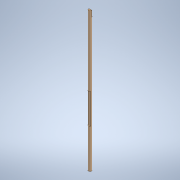
# Autodesk Inventor part: Wheel Shaft 125mm
Saved by Autodesk Inventor 2021.1 (Build 251245010, 245A)
## iProperties
Created: 2025-09-16
Material: Bronze, Soft Tin
Document SubType Name: Modeling
Designer: SD
Density: 8.874 g/cm^3
Appearance: Brindle
Mass: 8.09145 g
Surface Area: 13.019 cm^2
Volume: 0.911816 cm^3
Project: Automatic Tea Steeping mechanism
Part Number: Wheel Shaft 125mm
Length: 139.500 mm
BOM-Mass: 0.00809
BOM-Area: 0.001
Diameter: 3.000 mm
Author: SD
Title: Wheel Shaft 125mm
Autodesk Inventor part; units mm, degrees
ref_plane "YZ Plane" through (0, 0, 0) normal (1, 0, 0) x (0, 1, 0)
ref_plane "XZ Plane" through (0, 0, 0) normal (0, 1, 0) x (-1, 0, 0)
ref_plane "XY Plane" through (0, 0, 0) normal (0, 0, 1) x (1, 0, 0)
sketch "Sketch4" plane through (0, 0, 0) normal (0, 1, 0) x (-1, 0, 0)
  circle A0 centre (0, 0) radius 1.5
  constraints: 1 centre point, 1 coincident, 1 other
extrude "Extrusion2" add sketch "Sketch4" along normal mid plane 139.5
sketch "Sketch13" plane through (0, 0, 0) normal (1, 0, 0) x (0, 1, 0)
  line L0 (70.3754, -0.5) -> (63.75, -0.5)
  line L1 (63.75, -0.5) -> (63.75, -2.4686)
  line L2 (63.75, -2.4686) -> (70.3754, -2.4686)
  line L3 (70.3754, -2.4686) -> (70.3754, -0.5)
  line L4 (-69.75, -1.5) -> (69.75, -1.5) projected
  line L5 (69.75, -1.5) -> (69.75, 1.5) projected
  line L6 (-0.35, 2.5026) -> (-30.35, 2.5026)
  line L7 (-30.35, 2.5026) -> (-30.35, 0.5)
  line L8 (-30.35, 0.5) -> (-0.35, 0.5)
  line L9 (-0.35, 0.5) -> (-0.35, 2.5026)
  line L10 (-69.75, 1.5) -> (69.75, 1.5) projected
  line L11 (-69.75, 1.5) -> (-69.75, -1.5) projected
  point P0 (0, 0)
  point P1 (-0.35, 1.5)
  point P2 (-30.35, 1.5)
  point P3 (69.75, -0.5)
  point P4 (63.75, -1.5)
  dimension "d89" = 1
  dimension "d90" = 6
  dimension "d91" = 1
  dimension "d92" = 30
  dimension "d93" = 39.4
  constraints: 16 end point, 4 parallel, 2 horizontal, 2 perpendicular
  measures "d89" distance between parallel lines of L4 L0
  measures "d90" distance between parallel lines of L1 L5
  measures "d91" distance between parallel lines of L8 L10
  measures "d92" distance of L6.start L6.end
  measures "d93" distance between parallel lines of L11 L7
extrude "Extrusion9" cut sketch "Sketch13" against normal through all both and the other way through all contours L5 L4 L1 L0 | L9 L8 L7 L10
body "Solid2"
